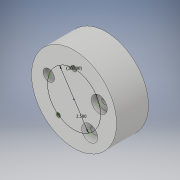
# Autodesk Inventor part: Hole Practice
Saved by Autodesk Inventor 2017 (Build 210142000, 142)
## iProperties
Created: 2020-03-03
Part Number: Hole Practice
Material: Generic
Document SubType Name: Modeling
Designer: 10042265
Density: 1 g/cm^3
Appearance: Default
Author: 10042265
Autodesk Inventor part; units mm, degrees
ref_plane "YZ Plane" through (0, 0, 0) normal (1, 0, 0) x (0, 1, 0)
ref_plane "XZ Plane" through (0, 0, 0) normal (0, 1, 0) x (-1, 0, 0)
ref_plane "XY Plane" through (0, 0, 0) normal (0, 0, 1) x (1, 0, 0)
sketch "Sketch1" plane through (0, 0, 0) normal (0, 0, 1) x (1, 0, 0)
  circle A0 centre (0, 0) radius 50.8
  constraints: 1 centre point, 1 coincident
extrude "Extrusion1" add sketch "Sketch1" along normal blind 38.1
sketch "Sketch2" plane through (0, 0, 38.1) normal (0, 0, 1) x (1, 0, 0)
  circle A0 centre (0, 0) radius 31.75 construction
  circle A1 centre (0, 0) radius 31.75 construction
  circle A2 centre (0, 0) radius 31.75 construction
  circle A3 centre (0, 0) radius 31.75 construction
  circle A4 centre (0, 0) radius 31.75 construction
  point P0 (0, 31.75)
  point P1 (-30.196, 9.8113)
  point P2 (-18.6622, -25.6863)
  point P3 (18.6622, -25.6863)
  point P4 (30.196, 9.8113)
  dimension "d8" = 63.5
  dimension "d11" = 360
  constraints: 3 coincident, 1 vertical alignment, 28 other
hole "Hole1" at (0, 31.75, 38.1) direction (0, 0, -1) diameter 6.35 depth 38.1 tip angle 118
hole "Hole2" at (30.196, 9.8113, 38.1) direction (0, 0, -1) diameter 6.985 depth 38.1 tip angle 118 counterbore diameter 19.05 counterbore depth 6.35
hole "Hole3" at (18.6622, -25.6863, 38.1) direction (0, 0, -1) diameter 9.0678 end through all countersink diameter 19.05 countersink angle 82
hole "Hole4" at (-18.6622, -25.6863, 38.1) direction (0, 0, -1) diameter 4.9784 end through all thread size "1/4-20 UNC" class "1B" standard "ANSI Unified Screw Threads"
hole "Hole5" at (-30.196, 9.8113, 38.1) direction (0, 0, -1) diameter 13.4874 end through all clearance for "Hex Head Bolt" size "1/2" standard "Ansi Unified Screw Threads"
body "Solid1"
